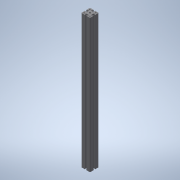
# Autodesk Inventor part: 6060-3.5
Saved by Autodesk Inventor 2022 (Build 260153000, 153)
## iProperties
Category: PARTsolutions
Company: MISUMI
Part Number: 6060-3.5
Material: Generic
Catalog Web Link: www.cadenas.de
Description: NFS8-6060, HFS8-6060, GFS8-6060, HFSF8-6060, HFST8-6060-HFS8 Series Aluminum Extrusions 60 Square -1 Slot-
Vendor: MISUMI
Document SubType Name: Modeling
Designer: partserver
Manufacturer: MISUMI
Mass: 2575.18 g
Surface Area: 5350.47 cm^2
Volume: 2575.18 cm^3
Density: 1 g/cm^3
Appearance: PSOLRGB-175-175-175
PSOL_IDENT_0: {$CADENAS_DATA\23d-libs\misumi\metric\38_al_extrusions_blackets\8_45\hfs8_6060.prj},592 {VTYP=3D},{N
PSOL_IDENT_1: B=GFS8-6060-1000},{LINA=GFS8-6060-1000},{NN=NFS8-6060, HFS8-6060, GFS8-6060, HFSF8-6060, HFST8-6060}
PSOL_IDENT_2: ,{DATE=17.06.2021 07:30:50},{GEOMDATE=08.06.2016 01:16:00},{VERSION=},{LINEID=80},{WBVAR=L,ALT1,ALT2
PSOL_IDENT_3: ,ALT4,ALT5,CP5,DL5,DR5,ALT6,ALT9,ALT10,ALT11,HP6,NHL6,DL6,NHR6,DR6,ALT7,ALT8,NH9,AH,BH,CH,DH,EH,NH10
PSOL_IDENT_4: ,AV,BV,CV,DV,EV,NH11,AP,BP,CP,DP,EP,ALT12,ALT13,Z,NH12,XA,XB,XC,XD,XE,NH13,YA,YB,YC,YD,YE,ALT14,HP14
PSOL_IDENT_5: ,DL14,DR14,ALT15,HP15,DL15,DR15,ALT16,HP16,DL16,DR16,ALT19,ALT20},{WBNUMERIC=L,NH9,AH,BH,CH,DH,EH,NH
PSOL_IDENT_6: 10,AV,BV,CV,DV,EV,NH11,AP,BP,CP,DP,EP,NH12,XA,XB,XC,XD,XE,NH13,YA,YB,YC,YD,YE}  {NB=GFS8-6060-1000},
PSOL_IDENT_7: {LINA=GFS8-6060-1000},{KT=DUMMY},{PN=GFS8-6060-1000},{TPS=GFS8-6060},{MAT=6061-T6 Aluminum Alloy Equ
PSOL_IDENT_8: ivalent},{ST=Clear Anodize},{FRMW=60},{FRMH=60},{FRD=10.5},{L=1000},{MASS=6.96},{SA=2577},{LX=79.86x
PSOL_IDENT_9: 10^4},{LY=79.86x10^4},{ALT1=},{M1=0},{IDM1=10.106},{DPL1=0},{DPR1=0},{ALT1PN=},{ALT2=},{ALT2ALG= '','
PSOL_IDENT_10: w/o End Tapping (Heli-Coil Insert)','LHP','with LHP (Tapping on the Left (Heli-Coil Insert))','RHP','
PSOL_IDENT_11: with RHP (Tapping on the Right (Heli-Coil Insert))','HPW','with HPW (Tapping on Both Ends (Heli-Coil
PSOL_IDENT_12: Insert))' },{M2=0},{DP2=0},{ALT2PN=},{ALT4=},{ALT4ALG= '', 'w/o SC (High Precision Cut)', 'SC', 'wi
PSOL_IDENT_13: th SC (High Precision Cut)' },{ALT4PN=},{ALT5=},{ALT5ALG= '','w/o 45 Degree Cut','1','with 45 Degree
PSOL_IDENT_14: Cut' },{CP5=},{CP5ALG= '','N/A' },{DL5=},{DL5ALG= '','N/A' },{DR5=},{DR5ALG= '','N/A' },{FRMLALT5=0
PSOL_IDENT_15: },{FRMRALT5=0},{ALT5PN=},{ALT6=},{ALT6ALG= '','w/o Fastening Location Wrench Access Hole Alterations'
PSOL_IDENT_16: ,'1','with Fastening Location Wrench Access Hole Alterations' },{ALT9=},{ALT9ALG= '','w/o Location S
PSOL_IDENT_17: pecified Wrench Access Hole Alteratons (Horizontal)','1','with Location Specified Wrench Access Hole
PSOL_IDENT_18: Alteratons (Horizontal)' },{ALT10=},{ALT10ALG= '','w/o Location Specified Wrench Access Hole Altera
PSOL_IDENT_19: tons (Vertical)','1','with Location Specified Wrench Access Hole Alteratons (Vertical)' },{ALT11=},{
PSOL_IDENT_20: ALT11ALG= '','w/o Location Specified Wrench Access Hole Alteratons (Crisscross)','1','with Location
PSOL_IDENT_21: Specified Wrench Access Hole Alteratons (Crisscross)' },{HP6=},{HP6ALG= '','N/A' },{NHL6=},{NHL6ALG=
PSOL_IDENT_22: '','N/A' },{DL6=},{DL6ALG= '','N/A' },{NHR6=},{NHR6ALG= '','N/A' },{DR6=},{DR6ALG= '','N/A' },{HL6=
PSOL_IDENT_23: 0.0},{HL6D=0.0},{HR6=0.0},{HR6D=0.0},{J6=0},{J6D=0},{K6=0},{K6D=0},{DD6=0},{DD6ALG=0},{ALT7=},{ALT7A
PSOL_IDENT_24: LG= '','N/A' },{ALT8=},{ALT8ALG= '','N/A' },{ALT678PN=},{NH9=0},{NH9MAX=5},{NH9ALG=[0]},{AH=0.0},{AH
PSOL_IDENT_25: MIN=7},{AHMAX=995},{AHALG=[0]},{BH=0.0},{BHMIN=2},{BHMAX=997},{BHALG=[0]},{CH=0.0},{CHMIN=2},{CHMAX=
PSOL_IDENT_26: 999},{CHALG=[0]},{DH=0.0},{DHMIN=2},{DHMAX=1001},{DHALG=[0]},{EH=0.0},{EHMIN=2},{EHMAX=993},{EHALG=[
PSOL_IDENT_27: 0]},{NH10=0},{NH10MAX=5},{NH10ALG=[0]},{AV=0.0},{AVMIN=7},{AVMAX=995},{AVALG=[0]},{BV=0.0},{BVMIN=2}
PSOL_IDENT_28: ,{BVMAX=997},{BVALG=[0]},{CV=0.0},{CVMIN=2},{CVMAX=999},{CVALG=[0]},{DV=0.0},{DVMIN=2},{DVMAX=1001},
PSOL_IDENT_29: {DVALG=[0]},{EV=0.0},{EVMIN=2},{EVMAX=993},{EVALG=[0]},{NH11=0},{NH11MAX=5},{NH11ALG=[0]},{AP=0.0},{
PSOL_IDENT_30: APMIN=7},{APMAX=995},{APALG=[0]},{BP=0.0},{BPMIN=2},{BPMAX=997},{BPALG=[0]},{CP=0.0},{CPMIN=2},{CPMA
PSOL_IDENT_31: X=999},{CPALG=[0]},{DP=0.0},{DPMIN=2},{DPMAX=1001},{DPALG=[0]},{EP=0.0},{EPMIN=2},{EPMAX=993},{EPALG=
PSOL_IDENT_32: [0]},{ALT9PN=},{ALT10PN=},{ALT11PN=},{ALT91011PN=},{ALT12=},{ALT12ALG= '','w/o Counterbore Hole in S
PSOL_IDENT_33: pecified Position (Vertical)','1','with Counterbore Hole in Specified Position (Vertical)' },{ALT13=
PSOL_IDENT_34: },{ALT13ALG= '','w/o Counterbore Hole in Specified Position (Horizontal)','1','with Counterbore Hole
PSOL_IDENT_35: in Specified Position (Horizontal)' },{Z=},{ZALG= '','N/A' },{DD12=0.0},{DD112=0.0},{NH12=0},{NH12M
PSOL_IDENT_36: AX=5},{NH12ALG=[0]},{XA=0.0},{XAMIN=7},{XAMAX=995},{XAALG=[0]},{XB=0.0},{XBMIN=2},{XBMAX=997},{XBALG=
PSOL_IDENT_37: [0]},{XC=0.0},{XCMIN=2},{XCMAX=999},{XCALG=[0]},{XD=0.0},{XDMIN=2},{XDMAX=1001},{XDALG=[0]},{XE=0.0}
PSOL_IDENT_38: ,{XEMIN=2},{XEMAX=993},{XEALG=[0]},{NH13=0},{NH13MAX=5},{NH13ALG=[0]},{YA=0.0},{YAMIN=7},{YAMAX=995}
PSOL_IDENT_39: ,{YAALG=[0]},{YB=0.0},{YBMIN=2},{YBMAX=997},{YBALG=[0]},{YC=0.0},{YCMIN=2},{YCMAX=999},{YCALG=[0]},{
PSOL_IDENT_40: YD=0.0},{YDMIN=2},{YDMAX=1001},{YDALG=[0]},{YE=0.0},{YEMIN=2},{YEMAX=993},{YEALG=[0]},{ALT12PN=},{AL
PSOL_IDENT_41: T13PN=},{ALT1213PN=},{ALT14=},{ALT14ALG= '','w/o D Type Hole Alteration','1','with D Type Hole Alter
PSOL_IDENT_42: ation' },{HP14=},{HP14ALG= '','N/A' },{DL14=},{DL14ALG= '','N/A' },{DR14=},{DR14ALG= '','N/A' },{H14=
PSOL_IDENT_43: 0.0},{D14=0.0},{ALT14PN=},{ALT15=},{ALT15ALG= '','w/o S Type Hole Alteration','1','with S Type Hole
PSOL_IDENT_44: Alteration' },{HP15=},{HP15ALG= '','N/A' },{DL15=},{DL15ALG= '','N/A' },{DR15=},{DR15ALG= '','N/A' }
PSOL_IDENT_45: ,{H15=0.0},{D115=0},{D215=0.0},{ALT15PN=},{ALT16=},{ALT16ALG= '','w/o M Type Hole Alteration','1','w
PSOL_IDENT_46: ith M Type Hole Alteration' },{HP16=},{HP16ALG= '','N/A' },{DL16=},{DL16ALG= '','N/A' },{DR16=},{DR1
PSOL_IDENT_47: 6ALG= '','N/A' },{H116=0},{D16=0.0},{ALT16PN=},{ALT19=},{ALT19ALG= '','w/o Hole Machining for End Pl
PSOL_IDENT_48: ate Mounting','LTS','with LTS (Hole Machining for End Plate Mounting)','RTS','with RTS (Hole Machini
PSOL_IDENT_49: ng for End Plate Mounting)','TSW','with TSW (Hole Machining for End Plate Mounting)' },{M19=0},{DP19=
PSOL_IDENT_50: 0},{ALT19PN=},{ALT20=},{ALT20PN=},{TFW=0},{TFH=0},{ERRORALT01=OK},{ERRORALT02=OK},{ERRORALT05=OK},{E
PSOL_IDENT_51: RRORALT06091=OK},{ERRORALT06092=OK},{ERRORALT06093=OK},{ERRORALT06094=OK},{ERRORALT06101=OK},{ERRORA
PSOL_IDENT_52: LT06102=OK},{ERRORALT06103=OK},{ERRORALT06104=OK},{ERRORALT06111=OK},{ERRORALT06112=OK},{ERRORALT061
PSOL_IDENT_53: 13=OK},{ERRORALT06114=OK},{ERRORALT06121=OK},{ERRORALT06122=OK},{ERRORALT06123=OK},{ERRORALT06124=OK
PSOL_IDENT_54: },{ERRORALT06131=OK},{ERRORALT06132=OK},{ERRORALT06133=OK},{ERRORALT06134=OK},{ERRORALT0614=OK},{ERR
PSOL_IDENT_55: ORALT0615=OK},{ERRORALT0616=OK},{ERRORALT0619=OK},{ERRORALT0911=OK},{ERRORALT0913=OK},{ERRORALT0914=
PSOL_IDENT_56: OK},{ERRORALT0915=OK},{ERRORALT0916=OK},{ERRORALT0919=OK},{ERRORALT1011=OK},{ERRORALT1012=OK},{ERROR
PSOL_IDENT_57: ALT1014=OK},{ERRORALT1015=OK},{ERRORALT1016=OK},{ERRORALT1019=OK},{ERRORALT1112=OK},{ERRORALT1113=OK
PSOL_IDENT_58: },{ERRORALT1114=OK},{ERRORALT1115=OK},{ERRORALT1116=OK},{ERRORALT1119=OK},{ERRORALT1214=OK},{ERRORAL
PSOL_IDENT_59: T1215=OK},{ERRORALT1216=OK},{ERRORALT1219=OK},{ERRORALT1314=OK},{ERRORALT1315=OK},{ERRORALT1316=OK},
PSOL_IDENT_60: {ERRORALT1319=OK},{ERRORALT1415=OK},{ERRORALT1416=OK},{ERRORALT1419=OK},{ERRORALT1516=OK},{ERRORALT1
PSOL_IDENT_61: 519=OK},{ERRORALT1619=OK},{ERRORPN=}
NB: GFS8-6060-1000
NN: NFS8-6060, HFS8-6060, GFS8-6060, HFSF8-6060, HFST8-6060
NT: HFS8 Series Aluminum Extrusions 60 Square -1 Slot-
NBSYN: $PN.
LINA: GFS8-6060-1000
CATALOG: Misumi
PN: GFS8-6060-1000
TPS: GFS8-6060
MAT: 6061-T6 Aluminum Alloy Equivalent
ST: Clear Anodize
L: 1000
MASS: 6.96
SA: 2577
LX: 79.86x10^4
LY: 79.86x10^4
ALT1: w/o End Tapping
M1: 0
DPL1: 0
DPR1: 0
ALT2: w/o End Tapping (Heli-Coil Insert)
M2: 0
DP2: 0
ALT4: w/o SC (High Precision Cut)
ALT5: w/o 45 Degree Cut
CP5: N/A
DL5: N/A
DR5: N/A
ALT6: w/o Fastening Location Wrench Access Hole Alterations
ALT9: w/o Location Specified Wrench Access Hole Alteratons (Horizontal)
ALT10: w/o Location Specified Wrench Access Hole Alteratons (Vertical)
ALT11: w/o Location Specified Wrench Access Hole Alteratons (Crisscross)
HP6: N/A
NHL6: N/A
DL6: N/A
NHR6: N/A
DR6: N/A
HL6D: 0
HR6D: 0
J6D: 0
K6D: 0
DD6: 0
ALT7: N/A
ALT8: N/A
NH9: 0
AH: 0
BH: 0
CH: 0
DH: 0
EH: 0
NH10: 0
AV: 0
BV: 0
CV: 0
DV: 0
EV: 0
NH11: 0
AP: 0
BP: 0
CP: 0
DP: 0
EP: 0
ALT12: w/o Counterbore Hole in Specified Position (Vertical)
ALT13: w/o Counterbore Hole in Specified Position (Horizontal)
Z: N/A
DD12: 0
DD112: 0
NH12: 0
XA: 0
XB: 0
XC: 0
XD: 0
XE: 0
NH13: 0
YA: 0
YB: 0
YC: 0
YD: 0
YE: 0
ALT14: w/o D Type Hole Alteration
HP14: N/A
DL14: N/A
DR14: N/A
H14: 0
D14: 0
ALT15: w/o S Type Hole Alteration
HP15: N/A
DL15: N/A
DR15: N/A
H15: 0
D115: 0
D215: 0
ALT16: w/o M Type Hole Alteration
HP16: N/A
DL16: N/A
DR16: N/A
H116: 0
D16: 0
ALT19: w/o Hole Machining for End Plate Mounting
M19: 0
DP19: 0
ALT20: w/o CW (End Face C Chamfering)
SUPPLIER: MISUMI
ARTICLENO: GFS8-6060-1000
BOMINFO: GFS8-6060-1000
CREATOR: CADENAS GmbH
Title: GFS8-6060-1000
Author: Cadenas PARTsolutions
Comments: HFS8 Series Aluminum Extrusions 60 Square -1 Slot-
Autodesk Inventor part; units mm, degrees
sketch "Sketch_60" plane through (0, 0, 0) normal (0, 0, 1) x (1, 0, 0)
  arc A0 (-30, -27) -> (-27, -30) centre (-27, -27) ccw
  line L0 (-27, -30) -> (-5, -30)
  line L1 (-5, -30) -> (-5, -24)
  line L2 (-5, -24) -> (-10, -24)
  line L3 (-10, -24) -> (-10, -19.6167)
  line L4 (-10, -19.6167) -> (-7.3833, -17)
  line L5 (-7.3833, -17) -> (-3.3464, -17)
  line L6 (-3.3464, -17) -> (-3, -16.8)
  line L7 (-3, -16.8) -> (-2.6536, -17)
  line L8 (-2.6536, -17) -> (-1.2124, -17)
  line L9 (-1.2124, -17) -> (0, -16.3)
  line L10 (0, -16.3) -> (1.2124, -17)
  line L11 (1.2124, -17) -> (2.6536, -17)
  line L12 (2.6536, -17) -> (3, -16.8)
  line L13 (3, -16.8) -> (3.3464, -17)
  line L14 (3.3464, -17) -> (7.3833, -17)
  line L15 (7.3833, -17) -> (10, -19.6167)
  line L16 (10, -19.6167) -> (10, -24)
  line L17 (10, -24) -> (5, -24)
  line L18 (5, -24) -> (5, -30)
  line L19 (5, -30) -> (27, -30)
  arc A1 (27, -30) -> (30, -27) centre (27, -27) ccw
  line L20 (30, -27) -> (30, -5)
  line L21 (30, -5) -> (24, -5)
  line L22 (24, -5) -> (24, -10)
  line L23 (24, -10) -> (19.6167, -10)
  line L24 (19.6167, -10) -> (17, -7.3833)
  line L25 (17, -7.3833) -> (17, -3.3464)
  line L26 (17, -3.3464) -> (16.8, -3)
  line L27 (16.8, -3) -> (17, -2.6536)
  line L28 (17, -2.6536) -> (17, -1.2124)
  line L29 (17, -1.2124) -> (16.3, 0)
  line L30 (16.3, 0) -> (17, 1.2124)
  line L31 (17, 1.2124) -> (17, 2.6536)
  line L32 (17, 2.6536) -> (16.8, 3)
  line L33 (16.8, 3) -> (17, 3.3464)
  line L34 (17, 3.3464) -> (17, 7.3833)
  line L35 (17, 7.3833) -> (19.6167, 10)
  line L36 (19.6167, 10) -> (24, 10)
  line L37 (24, 10) -> (24, 5)
  line L38 (24, 5) -> (30, 5)
  line L39 (30, 5) -> (30, 27)
  arc A2 (30, 27) -> (27, 30) centre (27, 27) ccw
  line L40 (27, 30) -> (5, 30)
  line L41 (5, 30) -> (5, 24)
  line L42 (5, 24) -> (10, 24)
  line L43 (10, 24) -> (10, 19.6167)
  line L44 (10, 19.6167) -> (7.3833, 17)
  line L45 (7.3833, 17) -> (3.3464, 17)
  line L46 (3.3464, 17) -> (3, 16.8)
  line L47 (3, 16.8) -> (2.6536, 17)
  line L48 (2.6536, 17) -> (1.2124, 17)
  line L49 (1.2124, 17) -> (0, 16.3)
  line L50 (0, 16.3) -> (-1.2124, 17)
  line L51 (-1.2124, 17) -> (-2.6536, 17)
  line L52 (-2.6536, 17) -> (-3, 16.8)
  line L53 (-3, 16.8) -> (-3.3464, 17)
  line L54 (-3.3464, 17) -> (-7.3833, 17)
  line L55 (-7.3833, 17) -> (-10, 19.6167)
  line L56 (-10, 19.6167) -> (-10, 24)
  line L57 (-10, 24) -> (-5, 24)
  line L58 (-5, 24) -> (-5, 30)
  line L59 (-5, 30) -> (-27, 30)
  arc A3 (-27, 30) -> (-30, 27) centre (-27, 27) ccw
  line L60 (-30, 27) -> (-30, 5)
  line L61 (-30, 5) -> (-24, 5)
  line L62 (-24, 5) -> (-24, 10)
  line L63 (-24, 10) -> (-19.6167, 10)
  line L64 (-19.6167, 10) -> (-17, 7.3833)
  line L65 (-17, 7.3833) -> (-17, 3.3464)
  line L66 (-17, 3.3464) -> (-16.8, 3)
  line L67 (-16.8, 3) -> (-17, 2.6536)
  line L68 (-17, 2.6536) -> (-17, 1.2124)
  line L69 (-17, 1.2124) -> (-16.3, 0)
  line L70 (-16.3, 0) -> (-17, -1.2124)
  line L71 (-17, -1.2124) -> (-17, -2.6536)
  line L72 (-17, -2.6536) -> (-16.8, -3)
  line L73 (-16.8, -3) -> (-17, -3.3464)
  line L74 (-17, -3.3464) -> (-17, -7.3833)
  line L75 (-17, -7.3833) -> (-19.6167, -10)
  line L76 (-19.6167, -10) -> (-24, -10)
  line L77 (-24, -10) -> (-24, -5)
  line L78 (-24, -5) -> (-30, -5)
  line L79 (-30, -5) -> (-30, -27)
  circle A4 centre (20, 20) radius 3.5
  circle A5 centre (20, -20) radius 3.5
  circle A6 centre (-20, 20) radius 3.5
  circle A7 centre (-20, -20) radius 3.5
  constraints: 160 end point, 8 centre point, 8 point on circle
extrude "Extrusion1" add sketch "Sketch_60" against normal blind 914.4
sketch "Sketch2" plane through (0, 0, -914.4) normal (0, 0, -1) x (-1, 0, 0)
  point P0 (0, 0)
hole "Hole1" at (0, 0, -914.4) direction (0, 0, 1) diameter 10.5 depth 1000
ref_plane "C1_XY" through (0, 0, 0) normal (0, 0, 1) x (1, 0, 0)
ref_plane "C1_YZ" through (0, 0, 0) normal (1, 0, 0) x (0, 1, 0)
ref_plane "C1_ZX" through (0, 0, 0) normal (0, 1, 0) x (0, 0, 1)
ref_plane "to_frame_cap1_XY" through (0, 0, 0) normal (0, 0, 1) x (1, 0, 0)
ref_plane "to_frame_cap1_YZ" through (0, 0, 0) normal (1, 0, 0) x (0, 1, 0)
ref_plane "to_frame_cap1_ZX" through (0, 0, 0) normal (0, 1, 0) x (0, 0, 1)
ref_plane "to_frame_cap2_XY" through (0, 0, -1000) normal (0, 0, -1) x (1, 0, 0)
ref_plane "to_frame_cap2_YZ" through (0, 0, -1000) normal (1, 0, 0) x (0, -1, 0)
ref_plane "to_frame_cap2_ZX" through (0, 0, -1000) normal (0, -1, 0) x (0, 0, -1)
body "Solid1"
